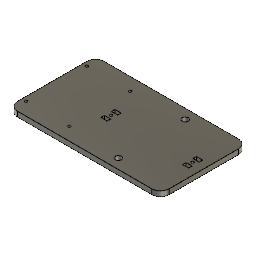
base v4 (Autodesk Fusion 360 design; units mm, degrees)
Autodesk Fusion 360 part; units mm, degrees
note: some values were not read from the file. Set by a fixed rule: which sketch regions a step uses.
sketch "Sketch1" plane through (0, 0, 0) normal (0, 0, 1) x (1, 0, 0)
  line L0 (10, 0) -> (165, 0)
  line L1 (175, 10) -> (175, 90)
  line L2 (165, 100) -> (10, 100)
  line L3 (0, 90) -> (0, 10)
  line L4 (5, 85) -> (55, 85)
  line L5 (55, 85) -> (55, 15)
  line L6 (55, 15) -> (5, 15)
  line L7 (5, 15) -> (5, 85)
  line L8 (5, 50) -> (0, 50)
  circle A0 centre (5, 85) radius 1.5
  circle A1 centre (55, 85) radius 1.5
  circle A2 centre (5, 15) radius 1.5
  circle A3 centre (55, 15) radius 1.5
  line L9 (55, 100) -> (55, 0)
  line L10 (65, 100) -> (65, 0)
  line L11 (165, 0) -> (165, 100)
  line L12 (65, 57.5) -> (71, 57.5)
  line L13 (71, 57.5) -> (71, 42.5)
  line L14 (71, 42.5) -> (65, 42.5)
  line L15 (65, 42.5) -> (65, 57.5)
  line L16 (65, 57.5) -> (71, 57.5)
  line L17 (71, 57.5) -> (71, 54.5)
  line L18 (71, 54.5) -> (65, 54.5)
  line L19 (65, 54.5) -> (65, 57.5)
  line L20 (71, 42.5) -> (65, 42.5)
  line L21 (65, 42.5) -> (65, 45.5)
  line L22 (65, 45.5) -> (71, 45.5)
  line L23 (71, 45.5) -> (71, 42.5)
  line L24 (65, 100) -> (165, 100)
  line L25 (115, 100) -> (115, 0)
  line L26 (159, 57.5) -> (159, 42.5)
  line L27 (159, 54.5) -> (165, 54.5)
  line L28 (165, 57.5) -> (159, 57.5)
  line L29 (165, 45.5) -> (159, 45.5)
  line L30 (159, 42.5) -> (165, 42.5)
  circle A4 centre (115, 88.5) radius 3.5
  circle A5 centre (115, 11.5) radius 3.5
  line L31 (115, 88.5) -> (115, 11.5)
  arc A6 (10, 100) -> (0, 90) centre (10, 90) ccw
  arc A7 (0, 10) -> (10, 0) centre (10, 10) ccw
  arc A8 (175, 90) -> (165, 100) centre (165, 90) ccw
  arc A9 (165, 0) -> (175, 10) centre (165, 10) ccw
  line L32 (64.5, 58) -> (71.5, 58)
  line L33 (71.5, 58) -> (71.5, 54)
  line L34 (71.5, 54) -> (64.5, 54)
  line L35 (64.5, 54) -> (64.5, 58)
  line L36 (71.5, 42) -> (64.5, 42)
  line L37 (64.5, 42) -> (64.5, 46)
  line L38 (64.5, 46) -> (71.5, 46)
  line L39 (71.5, 46) -> (71.5, 42)
  line L40 (159, 57.5) -> (165, 57.5)
  line L41 (165, 57.5) -> (165, 54.5)
  line L42 (165, 54.5) -> (159, 54.5)
  line L43 (159, 54.5) -> (159, 57.5)
  line L44 (159, 45.5) -> (165, 45.5)
  line L45 (165, 45.5) -> (165, 42.5)
  line L46 (165, 42.5) -> (159, 42.5)
  line L47 (159, 42.5) -> (159, 45.5)
  line L48 (158.5, 46) -> (165.5, 46)
  line L49 (165.5, 46) -> (165.5, 42)
  line L50 (165.5, 42) -> (158.5, 42)
  line L51 (158.5, 42) -> (158.5, 46)
  line L52 (158.5, 58) -> (165.5, 58)
  line L53 (165.5, 58) -> (165.5, 54)
  line L54 (165.5, 54) -> (158.5, 54)
  line L55 (158.5, 54) -> (158.5, 58)
  point P0 (0, 100)
  point P1 (65, 50)
  point P2 (65, 50)
  point P3 (115, 50)
  point P4 (115, 50)
  dimension "d1" = 50
  dimension "d2" = 70
  dimension "d3" = 100
  dimension "d4" = 90
  dimension "d5" = 5
  dimension "d6" = 3
  dimension "d7" = 3
  dimension "d8" = 3
  dimension "d9" = 3
  dimension "d11" = 120
  dimension "d12" = 10
  dimension "d13" = 10
  dimension "d14" = 6
  dimension "d15" = 15
  dimension "d16" = 3
  dimension "d17" = 3
  dimension "d18" = 77
  dimension "d19" = 7
  dimension "d20" = 7
  dimension "d21" = 10
  dimension "d22" = 10
  dimension "d23" = 10
  dimension "d24" = 10
  dimension "d27" = -0.5
  dimension "d28" = -0.5
  dimension "d29" = -0.5
  dimension "d30" = -0.5
  constraint horizontal L0
  constraint vertical L1
  constraint horizontal L2
  constraint vertical L3
  constraint horizontal L4
  constraint vertical L5
  constraint horizontal L6
  constraint vertical L7
  constraint midpoint L7 L8.start
  constraint coincident L4.start L7.end
  constraint coincident L4.end L5.start
  constraint coincident L6.end L7.start
  constraint coincident L5.end L6.start
  constraint coincident L0 L9.end
  constraint perpendicular L0 L9
  constraint coincident L2 L10.start
  constraint coincident L0 L10.end
  constraint perpendicular L0 L10
  constraint coincident L0 L11.start
  constraint coincident L2 L11.end
  constraint perpendicular L2 L11
  constraint coincident L4.end L9
  constraint horizontal L12
  constraint vertical L13
  constraint horizontal L14
  constraint vertical L15
  constraint horizontal L16
  constraint vertical L17
  constraint horizontal L18
  constraint vertical L19
  constraint coincident L13 L17.end
  constraint horizontal L20
  constraint vertical L21
  constraint horizontal L22
  constraint vertical L23
  constraint coincident L15 L21.end
  constraint midpoint L10 P2
  constraint midpoint L15 P2
  constraint coincident P2 P1
  constraint midpoint L24 L25.start
  constraint coincident L0 L25.end
  constraint perpendicular L0 L25
  constraint symmetric L12.start L25 L28.start
  constraint symmetric L12.end L25 L26.start
  constraint symmetric L13.end L25 L26.end
  constraint symmetric L17.end L25 L27.start
  constraint symmetric L18.end L25 L27.end
  constraint symmetric L14.end L25 L30.end
  constraint symmetric L21.end L25 L29.start
  constraint symmetric L22.end L25 L29.end
  constraint coincident L25 A4.centre
  constraint coincident L25 A5.centre
  constraint coincident A4.centre L31.start
  constraint coincident A5.centre L31.end
  constraint midpoint L31 P4
  constraint midpoint L25 P4
  constraint coincident P4 P3
  constraint coincident L3 L8.end
  constraint coincident P0 L2
  constraint coincident P0 L3
  constraint tangent L2 A6
  constraint tangent L3 A6
  constraint coincident origin L0
  constraint coincident origin L3
  constraint tangent L0 A7
  constraint tangent L3 A7
  constraint tangent L1 A8
  constraint tangent L2 A8
  constraint tangent L0 A9
  constraint tangent L1 A9
  constraint horizontal L40
  constraint vertical L41
  constraint horizontal L42
  constraint vertical L43
  constraint horizontal L44
  constraint vertical L45
  constraint horizontal L46
  constraint vertical L47
  measures "d1" distance of L4.start L4.end
  measures "d2" distance of L4.start L6.end
  measures "d3" distance of origin P0
  measures "d4" angle of L3 L8
  measures "d5" distance of L8.start L8.end
  measures "d6" diameter of A0
  measures "d7" diameter of A1
  measures "d8" diameter of A3
  measures "d9" diameter of A2
  measures "d11" distance of L1 L9
  measures "d12" distance of L9 L10
  measures "d13" distance of L1 L11
  measures "d14" distance of L12.start L12.end
  measures "d15" distance of L12.end L13.end
  measures "d16" distance of L16 L18
  measures "d17" distance of L14 L22
  measures "d18" distance of A4.centre A5.centre
  measures "d19" diameter of A4
  measures "d20" diameter of A5
  measures "d21" radius of A6
  measures "d22" radius of A7
  measures "d23" radius of A8
  measures "d24" radius of A9
extrude "Extrude1" add sketch "Sketch1" along normal blind 6 contours L0 L3 L6 L7 L8 A2 A3 L9 A7 | L0 L2 L5 A1 A3 L9 L10 L15 L32 L34 L35 L36 L37 L38 | L0 L2 L10 L13 L24 L25 A4 A5 L31 L32 L33 L34 L36 L38 L39 | L2 L3 L4 L7 L8 A0 A1 L9 A6 | L0 L2 L11 L24 L25 L26 A4 A5 L31 L48 L50 L51 L52 L54 L55 | L4 L5 L6 L7 A0 A1 A2 A3 L9 | L1 L11 A8 A9 L48 L49 L50 L52 L53 L54 | L10 L13 L15 L34 L38 | L11 L26 L48 L54
sketch "Sketch2" plane through (0, 0, 6) normal (0, 0, 1) x (-1, 0, 0)
  circle A0 centre (-5, -85) radius 1.5
  line L0 (-64.5, -46) -> (-71.5, -46)
  line L1 (-71.5, -46) -> (-71.5, -42)
  line L2 (-71.5, -42) -> (-64.5, -42)
  line L3 (-64.5, -42) -> (-64.5, -46)
  circle A1 centre (-55, -15) radius 1.5
  circle A2 centre (-5, -15) radius 1.5
  circle A3 centre (-115, -88.5) radius 3.5
  circle A4 centre (-55, -85) radius 1.5
  line L4 (-165.5, -54) -> (-158.5, -54)
  line L5 (-158.5, -54) -> (-158.5, -58)
  line L6 (-158.5, -58) -> (-165.5, -58)
  line L7 (-165.5, -58) -> (-165.5, -54)
  circle A5 centre (-115, -11.5) radius 3.5
  line L8 (-165.5, -42) -> (-158.5, -42)
  line L9 (-158.5, -42) -> (-158.5, -46)
  line L10 (-158.5, -46) -> (-165.5, -46)
  line L11 (-165.5, -46) -> (-165.5, -42)
  line L12 (-71.5, -54) -> (-64.5, -54)
  line L13 (-64.5, -54) -> (-64.5, -58)
  line L14 (-64.5, -58) -> (-71.5, -58)
  line L15 (-71.5, -58) -> (-71.5, -54)
  line L16 (-165, -100) -> (-10, -100)
  arc A6 (-10, -100) -> (0, -90) centre (-10, -90) ccw
  line L17 (0, -90) -> (0, -10)
  arc A7 (0, -10) -> (-10, 0) centre (-10, -10) ccw
  line L18 (-10, 0) -> (-165, 0)
  arc A8 (-165, 0) -> (-175, -10) centre (-165, -10) ccw
  line L19 (-175, -10) -> (-175, -90)
  arc A9 (-175, -90) -> (-165, -100) centre (-165, -90) ccw
  line L20 (-68, -54) -> (-68, -46)
  line L21 (-162, -54) -> (-162, -46)
  circle A10 centre (-162, -50) radius 1.5
  circle A11 centre (-68, -50) radius 1.5
  dimension "d31" = 3
  dimension "d32" = 3
  constraint midpoint L12 L20.start
  constraint midpoint L0 L20.end
  constraint midpoint L4 L21.start
  constraint midpoint L10 L21.end
  constraint midpoint L21 A10.centre
  constraint midpoint L20 A11.centre
  measures "d31" diameter of A11
  measures "d32" diameter of A10
extrude "Extrude2" cut sketch "Sketch2" against normal blind 10 contours L20 A11 | L20 A11 | L21 A10 | L21 A10
equation "d18 = ( ( 70 + 84 ) / 2 ) * 1 mm"
